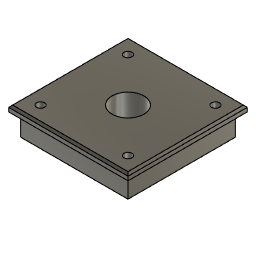
CAM-PoleMount-plug (Autodesk Fusion 360 design; units mm, degrees)
Autodesk Fusion 360 part; units mm, degrees
sketch "Sketch1" plane through (0, 0, 0) normal (0, 0, 1) x (1, 0, 0)
  line L0 (30, -30) -> (-30, -30)
  line L1 (-30, -30) -> (-30, 30)
  line L2 (-30, 30) -> (30, 30)
  line L3 (30, 30) -> (30, -30)
  line L4 (30, -30) -> (-30, 30) construction
  line L5 (-30, -30) -> (30, 30) construction
  circle A0 centre (0, 0) radius 8
  circle A1 centre (0, 0) radius 11
  line L6 (-27, -27) -> (-27, 27)
  line L7 (-27, 27) -> (27, 27)
  line L8 (27, 27) -> (27, -27)
  line L9 (27, -27) -> (-27, -27)
  circle A2 centre (22, -22) radius 2
  circle A3 centre (22, 22) radius 2
  circle A4 centre (-22, 22) radius 2
  circle A5 centre (-22, -22) radius 2
  line L10 (25, -25) -> (-25, -25)
  line L11 (-25, -25) -> (-25, 25)
  line L12 (-25, 25) -> (25, 25)
  line L13 (25, 25) -> (25, -25)
  circle A6 centre (0, 0) radius 24.25
  dimension "d1" = 60
  dimension "d2" = 60
  dimension "d3" = 16
  dimension "d4" = 3
  dimension "d5" = 3
  dimension "d6" = 4
  dimension "d8" = 8
  dimension "d10" = 360
  dimension "d11" = 5
  dimension "d31" = 48.5
  constraint horizontal L0
  constraint perpendicular L0 L1
  constraint parallel L0 L2
  constraint parallel L1 L3
  constraint coincident L4 A0.centre
  constraint coincident L5 A0.centre
  constraint coincident A0.centre A1.centre
  constraint coincident L4 A2.centre
  constraint concentric A0 A6
  measures "d1" distance of L1.end L2.end
  measures "d2" distance of L0.end L1.end
  measures "d3" diameter of A0
  measures "d6" diameter of A2
  measures "d8" distance of L0 A2.centre
  measures "d31" diameter of A6
extrude "Extrude5" add sketch "Sketch1" against normal blind 3 contours L0 L1 L2 L3
extrude "Extrude6" add sketch "Sketch1" against normal blind 15 contours L6 L7 L8 L9
extrude "Extrude7" add sketch "Sketch1" against normal blind 6 contours L10 L11 L12 L13 | A6
extrude "Extrude8" add sketch "Sketch1" against normal blind 20 contours A1
chamfer "Chamfer1" distance 1 angle 45 4 edges at (0, -30, 0) (30, 0, 0) (0, 30, 0) (-30, 0, 0)
chamfer "Chamfer2" distance 1 angle 45 4 edges at (0, -27, -15) (-27, 0, -15) (0, 27, -15) (27, 0, -15)
chamfer "Chamfer3" distance 1 angle 45 1 edges at (-7.4586, -2.8929, -20)
